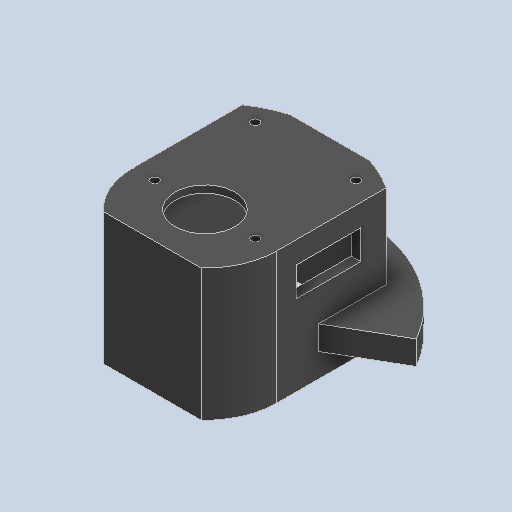
# Autodesk Inventor part: waist
Saved by Autodesk Inventor 2024.1 (Build 281209000, 209)
## iProperties
Created: 2024-02-14
Part Number: waist
Material: 一般
Document SubType Name: Modeling
Designer: hibik
Density: 1 g/cm^3
Appearance: 既定
Author: hibik
Autodesk Inventor part; units mm, degrees
ref_plane "YZ Plane" through (0, 0, 0) normal (1, 0, 0) x (0, 1, 0)
ref_plane "XZ Plane" through (0, 0, 0) normal (0, 1, 0) x (-1, 0, 0)
ref_plane "XY Plane" through (0, 0, 0) normal (0, 0, 1) x (1, 0, 0)
sketch "スケッチ1" plane through (0, 0, 0) normal (0, 1, 0) x (-1, 0, 0)
  line L0 (26, 0) -> (0, 0)
  line L1 (0, 0) -> (0, -33)
  line L2 (0, -33) -> (26, -33)
  line L3 (26, -33) -> (26, 0)
  line L4 (26, -9) -> (0, -9)
  line L5 (0, -9) -> (0, -33)
  line L6 (0, -33) -> (26, -33)
  line L7 (26, -33) -> (26, -9)
  circle A0 centre (13, -9) radius 13
  circle A1 centre (13, -9) radius 6.25
  circle A2 centre (13, -9) radius 27.2947
  circle A3 centre (13, -9) radius 32.2947
  circle A4 centre (13, -9) radius 15
  line L8 (28, -9) -> (-2, -9)
  line L9 (-2, -9) -> (-2, -35)
  line L10 (-2, -35) -> (28, -35)
  line L11 (28, -35) -> (28, -9)
  line L12 (23.198, 2) -> (2.802, 2)
  line L13 (13, -9) -> (40.968, -25.1473)
  line L14 (13, -9) -> (-14.968, -25.1473)
  point P0 (22.3808, 0)
  point P1 (3.6192, 0)
  point P2 (0, -9)
  point P3 (-17.3636, 2)
  point P4 (43.3636, 2)
  point P5 (25, 0)
  point P6 (26, -1.5167)
  point P7 (0, -1.5167)
  point P8 (1, 0)
  point P9 (21.3066, -35)
  point P10 (4.6934, -35)
  point P11 (0, -16.4833)
  point P12 (26, -16.4833)
  point P13 (0, -9)
  point P14 (26, -9)
  point P15 (28, -17.6603)
  point P16 (-2, -17.6603)
  point P17 (28, -31.8035)
  point P18 (-2, -31.8035)
  dimension "d0" = 26
  dimension "d1" = 33
  dimension "d2" = 24
  dimension "d3" = 12.5
  dimension "d6" = 5
  dimension "d7" = 2
  dimension "d8" = 2
  dimension "d9" = 2
  dimension "d16" = 60
  dimension "d17" = 60
  constraints: 30 end point, 7 parallel, 7 point on circle, 5 coincident, 4 centre point, 3 horizontal, 3 perpendicular, 2 midpoint, 1 point on line, 1 tangent, 3 other
  measures "d0" distance of L0.start L0.end
  measures "d1" distance of L2.end L0.start
  measures "d2" distance between parallel lines of L2 L4
  measures "d3" diameter of A1
  measures "d7" distance between parallel lines of L11 L3
  measures "d8" distance between parallel lines of L10 L6
  measures "d9" distance between parallel lines of L12 L0
  measures "d16" angle of L9 L14
  measures "d17" angle of L11 L13
extrude "押し出し1" add sketch "スケッチ1" against normal blind 1.5 contours A0 L4 A1 L0 | A0 L13 A1 L4 | L3 A4 L13 A0 | L3 L13 A4 | L13 A4 L14 A0 | A0 L14 A1 L13 | A0 L14 A4 L1 | L4 A1 L14 A0 | L3 L2 L1 L14 A4 L13 | A4 L14 L1
extrude "押し出し2" add sketch "スケッチ1" against normal blind 27.5 contours A4 L3 A0 L0 | L0 A0 L12 A4 | A4 L8 L3 | L0 A0 L12 | L8 A4 L3 | L11 L13 L3 A4 | A0 L1 A4 L0 | L0 A4 L12 A0 | L11 A2 L3 L13 | L8 A4 L1 | L1 A4 L8 | L1 L14 L9 A4 | A2 L10 L2 | L1 A2 L9 L14
extrude "押し出し3" add sketch "スケッチ1" against normal blind 22.5 contours L13 A2 L11 | L11 L10 A2 | A2 L13 A3 L14 L9 L10 L11 | L9 A2 L14 | A2 L10 L9 | A2 L10
extrude "押し出し4" cut sketch "スケッチ1" against normal blind 17.5 contours L13 A2 L11 | L11 L10 A2 | A2 L13 A3 L14 L9 L10 L11 | L9 A2 L14 | A2 L10 L9 | A2 L10
sketch "スケッチ2" plane through (2, -27.5, -9) normal (1, 0, 0) x (0, 0, -1)
  line L0 (17.5, 16.8) -> (4, 16.8) projected
  line L1 (4, 16.8) -> (4, 18.5) projected
  line L2 (4, 18.5) -> (0, 18.5) projected
  line L3 (0, 12.5) -> (0, 18.5) projected
  line L4 (0, 12.5) -> (21, 12.5) projected
  line L5 (21, 12.5) -> (21, 18.5) projected
  line L6 (21, 18.5) -> (17.5, 18.5) projected
  line L7 (17.5, 18.5) -> (17.5, 16.8) projected
  line L8 (4, 22.9122) -> (17.5, 22.9122) projected
  line L9 (17.5, 22.9122) -> (17.5, 19) projected
  line L10 (17.5, 19) -> (21, 19) projected
  line L11 (21, 19) -> (21, 26) projected
  line L12 (21, 26) -> (0, 26) projected
  line L13 (0, 19) -> (0, 26) projected
  line L14 (0, 19) -> (4, 19) projected
  line L15 (4, 19) -> (4, 22.9122) projected
  line L16 (4, 16.8) -> (17.5, 16.8)
  line L17 (17.5, 16.8) -> (17.5, 22.9122)
  line L18 (17.5, 22.9122) -> (4, 22.9122)
  line L19 (4, 22.9122) -> (4, 16.8)
  point P0 (-9, 27.5)
  point P1 (4, 19)
  point P2 (4, 18.5)
  constraints: 8 end point, 2 parallel, 1 horizontal, 1 perpendicular
extrude "押し出し5" cut sketch "スケッチ2" against normal up to surface (2 mm away) contours L0 L1 L19 L15 L8 L9 L17 L7
sketch "スケッチ3" plane through (0, 0, 0) normal (0, 1, 0) x (1, 0, 0)
  circle A0 centre (-2.5, 30) radius 0.85 projected
  circle A1 centre (-23.5, 30) radius 0.85 projected
  circle A2 centre (-23.5, 9) radius 0.85 projected
  circle A3 centre (-2.5, 9) radius 0.85 projected
  point P0 (0, 0)
extrude "押し出し6" cut sketch "スケッチ3" against normal blind 10
equation "\"d17\" = d16"
